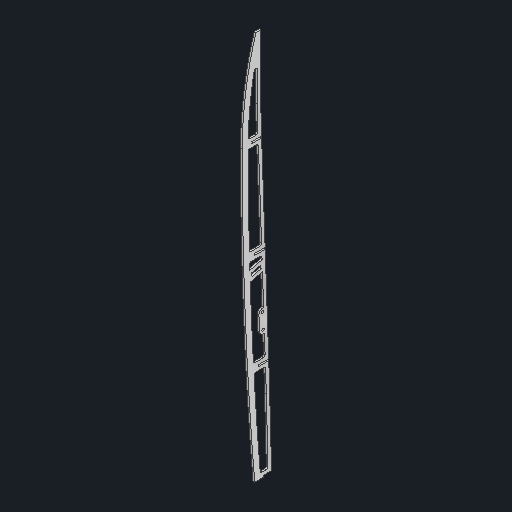
# Autodesk Inventor part: stringer_cowl
Saved by Autodesk Inventor 2023 (Build 270158030, 158C)
## iProperties
Created: 2022-03-23
Part Number: stringer_cowl
Material: Generic
Document SubType Name: Modeling
Designer: kardo
Density: 1 g/cm^3
Appearance: Default
Author: kardo
Autodesk Inventor part; units mm, degrees
ref_plane "YZ Plane" through (0, 0, 0) normal (1, 0, 0) x (0, 1, 0)
ref_plane "XZ Plane" through (0, 0, 0) normal (0, 1, 0) x (-1, 0, 0)
ref_plane "XY Plane" through (0, 0, 0) normal (0, 0, 1) x (1, 0, 0)
derived "parameters_frame.ipt"
derived "surface_body.ipt"
sketch "sk_rail_top_cowl" plane through (54.6, 0, 0) normal (1, 0, 0) x (0, 1, 0)
  spline S0 degree 2 poles (-345, 39.712) (-172.656, 54.3934) (0, 54.4) knots 0 0 0 1 1 1
  spline S1 degree 3 poles (0, 54.4) (37.026, 54.4) (80.784, 47.9917) (112.2, 37.536) knots 1 1 1 1 2 2 2 2
  point P0 (0, 0)
sketch "sk_rail_bottom_standoff" plane through (34.32, 0, 0) normal (1, 0, 0) x (0, 1, 0)
  line L0 (-345, 16.32) -> (-262.2001, 18.586)
  arc A0 (-262.2001, 18.586) -> (-241.5001, 19.2432) centre (-326.8578, 2381.2399) ccw
  line L1 (36.465, 28.832) -> (112.2, 28.832)
  arc A1 (36.465, 28.832) -> (11.22, 28.376) centre (36.465, -670.197) ccw
  line L2 (-241.5001, 19.2432) -> (11.22, 28.376)
  line L3 (-465, 0) -> (375, 0) construction
  line L4 (11.22, 28.376) -> (11.22, 0) construction
  line L5 (-241.5001, 19.2432) -> (-241.5001, 0) construction
  point P0 (0, 0)
  point P1 (-241.5001, 19.1524)
  point P2 (11.22, 28.832)
ref_plane "plane_middle" through (0, 0, 0) normal (0, 1, 0) x (-1, 0, 0)
ref_plane "plane_rear" through (0, -345, 0) normal (0, 1, 0) x (-1, 0, 0)
ref_plane "plane_cowl_right" through (54.6, 0, 0) normal (1, 0, 0) x (0, 1, 0)
ref_plane "plane_nose" through (0, 112.2, 0) normal (0, 1, 0) x (-1, 0, 0)
ref_plane "plane_tail_1" through (0, -114.9999, 0) normal (0, 1, 0) x (-1, 0, 0)
ref_plane "plane_tail_2" through (0, -230.0001, 0) normal (0, 1, 0) x (-1, 0, 0)
derived "stencil_frame.ipt"
sketch "sk_cowl_joint_locations" plane through (54.6, 0, 0) normal (1, 0, 0) x (0, 1, 0)
  line L0 (-345, 16.32) -> (-262.2001, 18.586) construction
  arc A0 (-262.2001, 18.586) -> (-241.5001, 19.2432) centre (-326.8578, 2381.2399) ccw construction
  line L1 (-241.5001, 19.2432) -> (11.22, 28.376) construction
  arc A1 (36.465, 28.832) -> (11.22, 28.376) centre (36.465, -670.197) ccw construction
  line L2 (36.465, 28.832) -> (112.2, 28.832) construction
  line L3 (94.8, 30.032) -> (36.465, 30.032) construction
  arc A2 (36.465, 30.032) -> (11.1767, 29.5752) centre (36.465, -670.197) ccw construction
  line L4 (11.1767, 29.5752) -> (-241.5434, 20.4424) construction
  arc A3 (-262.2329, 19.7855) -> (-241.5434, 20.4424) centre (-326.8578, 2381.2399) ccw construction
  line L5 (-262.2329, 19.7855) -> (-345, 17.5204) construction
  line L6 (-230.0001, 3089.1136) -> (-230.0001, -1866.0023) construction
  line L7 (-114.9999, 3089.1136) -> (-114.9999, -1866.0023) construction
  line L8 (-345, 3089.1136) -> (-345, -1866.0023) construction
  line L9 (0, 3089.1136) -> (0, -1866.0023) construction
  line L10 (-230.0001, 45.0685) -> (-230.0001, 20.8596) construction
  line L11 (-114.9999, 49.9659) -> (-114.9999, 25.0155) construction
  line L12 (-345, 17.5204) -> (-345, 17.5204)
  line L13 (-345, 17.5204) -> (-345, 36.9221) construction
  line L14 (-869.78, 3004.1953) -> (348.339, -1881.413) construction
  line L15 (-344.7623, 36.9221) -> (-345, 39.712) construction
  spline S0 degree 2 poles (-345, 39.712) (-172.656, 54.3934) (0, 54.4) knots 0 0 0 1 1 1
  spline S1 degree 3 poles (0, 54.4) (37.026, 54.4) (80.784, 47.9917) (112.2, 37.536) knots 1 1 1 1 2 2 2 2
  line L16 (0, 51.6) -> (0, 29.1713) construction
  spline S2 degree 3 poles (111.3158, 34.8793) (106.1488, 36.5989) (96.4909, 39.4217) (84.5445, 42.2265) (75.2974, 44.1359) (69.0059, 45.3094) (61.0256, 46.6466) (54.5653, 47.6105) (46.4371, 48.6777) (39.9092, 49.4192) (31.7597, 50.2005) (25.2653, 50.7072) (17.2211, 51.1873) (9.2717, 51.5118) (3.0586, 51.6) (0, 51.6) knots 1 1 1 1 1.166667 1.291667 1.333333 1.416667 1.458333 1.541667 1.583333 1.666667 1.708333 1.791667 1.833333 1.916667 2 2 2 2
  spline S3 degree 3 poles (0, 51.6) (-19.1708, 51.5993) (-52.7146, 51.3604) (-91.0402, 50.6121) (-119.7801, 49.8472) (-138.9379, 49.2354) (-162.8824, 48.3434) (-182.0358, 47.528) (-205.975, 46.3814) (-225.1241, 45.3623) (-249.0578, 43.9611) (-268.2026, 42.7383) (-292.131, 41.0825) (-316.0566, 39.2994) (-335.1942, 37.7372) (-344.7623, 36.9221) knots 0 0 0 0 0.166667 0.291667 0.333333 0.416667 0.458333 0.541666 0.583333 0.666666 0.708333 0.791666 0.833333 0.916666 1 1 1 1
  line L17 (-136.2088, 45.4676) -> (-130.9657, 24.4385) construction
  line L18 (-128.3953, 30.6635) -> (-132.2764, 29.6958) construction
  line L19 (-131.0168, 41.178) -> (-134.898, 40.2103) construction
  line L20 (-136.2088, 45.4676) -> (-132.3276, 46.4353) construction
  line L21 (-130.9657, 24.4385) -> (-127.0845, 25.4062) construction
  line L22 (-132.3276, 46.4353) -> (-132.5171, 52.2322) construction
  point P0 (0, 0)
  point P1 (-345, 27.2213)
  point P2 (-230.0001, 32.964)
  point P3 (-114.9999, 37.4907)
  point P4 (0, 40.3857)
  point P5 (-869.78, 3004.1953)
  point P6 (348.339, -1881.413)
  point P7 (-85.2629, 50.788)
  point P8 (0, 40.3857)
sketch "sk_servo_mount" plane through (-54.6, 0, 0) normal (1, 0, 0) x (0, 1, 0)
  line L0 (-241.5001, 19.2432) -> (11.22, 28.376) construction
  line L1 (-345, 3089.1136) -> (-345, -1866.0023) construction
  line L2 (0, 3089.1136) -> (0, -1866.0023) construction
  line L3 (-195.0558, 20.9216) -> (-195.2941, 27.5173) construction
  line L4 (-195.2941, 27.5173) -> (-177.3059, 28.1674) construction
  line L5 (-177.3059, 28.1674) -> (-177.0675, 21.5717) construction
  point P0 (0, 0)
  point P1 (-186.3, 27.8423)
sketch "sk_base" plane through (54.6, 0, 0) normal (1, 0, 0) x (0, 1, 0)
  line L0 (-345, 16.32) -> (-262.2001, 18.586) construction
  arc A0 (-262.2001, 18.586) -> (-241.5001, 19.2432) centre (-326.8578, 2381.2399) ccw construction
  line L1 (-241.5001, 19.2432) -> (11.22, 28.376) construction
  arc A1 (36.465, 28.832) -> (11.22, 28.376) centre (36.465, -670.197) ccw construction
  line L2 (36.465, 28.832) -> (112.2, 28.832) construction
  spline S0 degree 3 poles (0, 54.4) (37.026, 54.4) (80.784, 47.9917) (112.2, 37.536) knots 1 1 1 1 2 2 2 2 construction
  spline S1 degree 2 poles (-345, 39.712) (-172.656, 54.3934) (0, 54.4) knots 0 0 0 1 1 1 construction
  line L3 (-345, 4592.9714) -> (-345, -1605.7041) projected
  line L4 (112.2, 4592.9714) -> (112.2, -1605.7041) construction
  line L5 (110.2, 30.032) -> (36.465, 30.032)
  arc A2 (36.465, 30.032) -> (11.1767, 29.5752) centre (36.465, -670.197) ccw
  line L6 (11.1767, 29.5752) -> (-241.5434, 20.4424)
  arc A3 (-262.2329, 19.7855) -> (-241.5434, 20.4424) centre (-326.8578, 2381.2399) ccw
  line L7 (-262.2329, 19.7855) -> (-345.0328, 17.5196)
  line L8 (110.2, 35.668) -> (110.2, 30.032)
  line L9 (-345, 39.712) -> (-344.7963, 37.3207) construction
  line L10 (-344.7963, 37.3207) -> (-345, 37.3033)
  spline S2 degree 4 poles (-344.7963, 37.3207) (-258.8046, 44.646) (-172.6063, 49.5475) (-86.303, 51.9967) (0.0001, 52) knots 0 0 0 0 0 1 1 1 1 1
  spline S3 degree 5 poles (0, 52) (11.6151, 51.9997) (23.2289, 51.4722) (34.8145, 50.543) (57.0458, 48.0136) (79.0573, 44.0004) (89.562, 41.7015) (99.982, 38.9984) (110.2, 35.6678) knots 0 0 0 0 0 0 0.519409 0.519409 0.519409 1 1 1 1 1 1
  point P0 (0, 0)
  point P1 (-345, 17.5204)
  dimension "d3" = 2.4
  dimension "d2" = 1.2
  dimension "d4" = 2
  constraints: 12 end point, 4 point on circle, 2 centre point, 1 parallel, 1 perpendicular, 1 point on line, 12 other
  measures "d2" distance between parallel lines of L1 L6
  measures "d4" distance between parallel lines of L4 L8
extrude "thicken" add sketch "sk_base" along normal blind 2
sketch "sk_cut_weight" plane through (54.6, 0, 0) normal (1, 0, 0) x (0, 1, 0)
  spline S0 degree 3 poles (-344.7963, 37.3207) (-335.2272, 38.1358) (-316.0877, 39.6982) (-292.1597, 41.4815) (-268.2291, 43.1374) (-249.0824, 44.3603) (-225.1463, 45.7617) (-205.9953, 46.7809) (-182.0538, 47.9276) (-162.8984, 48.7431) (-138.9516, 49.6352) (-119.7919, 50.247) (-95.8396, 50.8845) (-76.6756, 51.2926) (-52.7179, 51.6755) (-28.7575, 51.931) (-9.5863, 51.9996) (0, 52) knots 0 0 0 0 0.083333 0.166667 0.208333 0.291667 0.333333 0.416667 0.458333 0.541667 0.583333 0.666667 0.708333 0.791667 0.833333 0.916667 1 1 1 1 construction
  line L0 (-262.2329, 19.7855) -> (-345.0328, 17.5196) construction
  line L1 (110.2, 35.668) -> (110.2, 30.032) construction
  line L2 (-114.9999, 4592.9714) -> (-114.9999, -1605.7041) construction
  line L3 (-230.0001, 4592.9714) -> (-230.0001, -1605.7041) construction
  line L4 (-345, 4592.9714) -> (-345, -1605.7041) construction
  line L5 (0, 4592.9714) -> (0, -1605.7041) construction
  line L6 (11.1767, 29.5752) -> (-241.5434, 20.4424) construction
  arc A0 (-262.2329, 19.7855) -> (-241.5434, 20.4424) centre (-326.8578, 2381.2399) ccw construction
  line L7 (110.2, 30.032) -> (36.465, 30.032) construction
  arc A1 (36.465, 30.032) -> (11.1767, 29.5752) centre (36.465, -670.197) ccw construction
  spline S1 degree 3 poles (0, 52) (3.0219, 52) (9.1586, 51.914) (17.0078, 51.5976) (24.9501, 51.1295) (31.3623, 50.6354) (39.4099, 49.8733) (45.8578, 49.1499) (53.8895, 48.1087) (60.2761, 47.168) (68.1706, 45.8627) (74.3991, 44.7169) (82.0351, 43.1629) (88.0081, 41.8244) (95.2639, 40.0376) (102.2888, 38.1399) (107.6186, 36.5095) (110.2, 35.668) knots 1 1 1 1 1.082229 1.164457 1.205571 1.2878 1.328914 1.411142 1.452257 1.534485 1.575599 1.657828 1.698942 1.78117 1.822284 1.904513 1.986741 1.986741 1.986741 1.986741 construction
  line L8 (-343, 17.5196) -> (-343, 52) construction
  line L9 (-228.0001, 52) -> (-228.0001, 17.5196) construction
  line L10 (-112.9999, 52) -> (-112.9999, 17.5196) construction
  line L11 (2, 52) -> (2, 17.5196) construction
  line L12 (-339, 30.7857) -> (-339, 21.6861)
  line L13 (-234.0001, 24.7176) -> (-234.0001, 38.2283)
  line L14 (-224.0001, 38.7947) -> (-224.0001, 25.079)
  line L15 (-108.9999, 43.5294) -> (-108.9999, 29.2349)
  line L16 (-4, 33.0294) -> (-4, 44.9979)
  line L17 (6, 44.9437) -> (6, 33.3908)
  line L18 (90.3642, 34.032) -> (36.465, 34.032)
  arc A2 (36.465, 34.032) -> (11.0322, 33.5726) centre (36.465, -670.197) ccw
  line L19 (11.0322, 33.5726) -> (-241.6879, 24.4398)
  arc A3 (-262.3423, 23.784) -> (-241.6879, 24.4398) centre (-326.8578, 2381.2399) ccw
  line L20 (-262.3423, 23.784) -> (-343, 21.5767)
  line L21 (-118.9999, 43.2475) -> (-118.9999, 28.8735)
  spline S2 degree 5 poles (90.3642, 34.0321) (83.5768, 35.7135) (76.7406, 37.198) (69.8723, 38.519) (51.8764, 41.5622) (33.7339, 43.6027) (22.5075, 44.4934) (11.2545, 44.9997) (0, 45) knots 0 0 0 0 0 0 0.383219 0.383219 0.383219 1 1 1 1 1 1
  spline S3 degree 4 poles (0.0003, 45) (-85.8525, 44.9967) (-171.7055, 42.5688) (-257.4548, 37.7099) (-343, 30.4481) knots 0 0 0 0 0 1 1 1 1 1
  point P0 (0, 0)
  dimension "d51" = 7
  dimension "d18" = 2
  dimension "d19" = 2
  dimension "d20" = 2
  dimension "d21" = 2
  dimension "d22" = 4
  dimension "d23" = 4
  dimension "d26" = 4
  dimension "d27" = 4
  dimension "d28" = 4
  dimension "d29" = 4
  dimension "d30" = 4
  dimension "d52" = 4
  constraints: 28 end point, 11 parallel, 9 point on line, 8 horizontal alignment, 4 point on circle, 2 centre point, 17 other
  measures "d18" distance between parallel lines of L3 L9
  measures "d19" distance between parallel lines of L10 L2
  measures "d20" distance between parallel lines of L11 L5
  measures "d21" distance between parallel lines of L8 L4
  measures "d22" distance between parallel lines of L8 L12
  measures "d23" distance between parallel lines of L13 L3
  measures "d26" distance between parallel lines of L9 L14
  measures "d27" distance between parallel lines of L10 L15
  measures "d28" distance between parallel lines of L16 L5
  measures "d29" distance between parallel lines of L11 L17
  measures "d30" distance between parallel lines of L21 L2
  measures "d52" distance between parallel lines of L7 L18
extrude "cut_weight" cut sketch "sk_cut_weight" along normal through all both and the other way through all contours S3 L13 L19 A3 L20 L12 | S3 L21 L19 L14 | S3 L16 L19 L15 | L17 S2 L18 A2 L19
fillet "rounding" radius 2 15 edges at (55.6, -234.0001, 24.7176) (55.6, -118.9999, 28.8735) (55.6, -4, 33.0294) (55.6, 6, 33.3908) (55.6, -108.9999, 29.2349) (55.6, -224.0001, 25.079) (55.6, -339, 21.6861) (55.6, -339, 30.7857) (55.6, -224.0001, 38.7947) (55.6, -108.9999, 43.5294) (55.6, 6, 44.9437) (55.6, -4, 44.9979) (55.6, -118.9999, 43.2475) (55.6, -234.0001, 38.2283) (55.6, 90.3642, 34.032)
sketch "sk_joint_motor_mount" plane through (54.6, 0, 0) normal (1, 0, 0) x (0, 1, 0)
  spline S0 degree 3 poles (-344.7963, 37.3207) (-335.2272, 38.1358) (-316.0877, 39.6982) (-292.1597, 41.4815) (-268.2291, 43.1374) (-249.0824, 44.3603) (-225.1463, 45.7617) (-205.9953, 46.7809) (-182.0538, 47.9276) (-162.8984, 48.7431) (-138.9516, 49.6352) (-119.7919, 50.247) (-95.8396, 50.8845) (-76.6756, 51.2926) (-52.7179, 51.6755) (-28.7575, 51.931) (-9.5863, 51.9996) (0, 52) knots 0 0 0 0 0.083333 0.166667 0.208333 0.291667 0.333333 0.416667 0.458333 0.541667 0.583333 0.666667 0.708333 0.791667 0.833333 0.916667 1 1 1 1 projected
  line L0 (11.1767, 29.5752) -> (-241.5434, 20.4424) projected
  line L1 (-131.0168, 41.178) -> (-128.3953, 30.6635) construction
  line L2 (-131.0168, 41.178) -> (-134.898, 40.2103) construction
  line L3 (-134.898, 40.2103) -> (-132.2764, 29.6958) construction
  line L4 (-132.2764, 29.6958) -> (-128.3953, 30.6635) construction
  line L5 (-141.3448, 49.5326) -> (-135.0513, 24.2908)
  line L6 (-129.0795, 49.9419) -> (-122.7944, 24.7338)
  point P0 (0, 0)
  dimension "d33" = 4
  dimension "d34" = 4
  dimension "d35" = 4
  constraints: 12 end point, 3 parallel, 2 coincident, 2 perpendicular, 2 point on line, 2 other
  measures "d33" distance between parallel lines of L1 L3
  measures "d34" distance between parallel lines of L3 L5
  measures "d35" distance between parallel lines of L1 L6
extrude "joint_motor_mount" add sketch "sk_joint_motor_mount" along normal blind 2
sketch "sk_joint_servo" plane through (54.6, 0, 0) normal (1, 0, 0) x (0, 1, 0)
  line L0 (11.1767, 29.5752) -> (-241.5434, 20.4424) projected
  line L1 (-171.8973, 22.9593) -> (-173.1987, 29.0456)
  arc A0 (-173.1987, 29.0456) -> (-177.4576, 32.3646) centre (-177.3059, 28.1674) ccw
  line L2 (-177.4576, 32.3646) -> (-195.4458, 31.7146)
  arc A1 (-195.4458, 31.7146) -> (-199.454, 28.0968) centre (-195.2941, 27.5173) ccw
  line L3 (-199.454, 28.0968) -> (-200.3127, 21.9324)
  point P0 (0, 0)
  dimension "d39" = 80
  dimension "d40" = 80
  dimension "d41" = 4.2
  constraints: 6 end point, 4 point on circle, 4 tangent, 2 centre point, 2 coincident, 2 point on line, 1 equal radius
  measures "d39" angle of L1 L0
  measures "d40" angle of L0 L3
  measures "d41" radius of A0
extrude "joint_servo" add sketch "sk_joint_servo" along normal blind 2
hole "drill_joint_servo" at (54.6, -195.2941, 27.5173) at (54.6, -177.3059, 28.1674) direction (1, 0, 0) diameter 3 end through all
sketch "sk_cowl_joint_cuts" plane through (54.6, 0, 0) normal (1, 0, 0) x (0, 1, 0)
  line L0 (-230.0001, 2991.5273) -> (-230.0001, -1280.4843) projected
  line L1 (-114.9999, 2991.5273) -> (-114.9999, -1280.4843) projected
  line L2 (0, 2991.5273) -> (0, -1280.4843) projected
  line L3 (-345, 2991.5273) -> (-345, -1280.4843) projected
  line L4 (-114.9999, -12.5093) -> (-112.9999, -12.5093)
  line L5 (-112.9999, -12.5093) -> (-112.9999, 37.4907)
  line L6 (-112.9999, 37.4907) -> (-114.9999, 37.4907)
  line L7 (0, -9.6143) -> (2, -9.6143)
  line L8 (2, -9.6143) -> (2, 40.3857)
  line L9 (2, 40.3857) -> (0, 40.3857)
  line L10 (-230.0001, 32.964) -> (-228.0001, 32.964)
  line L11 (-228.0001, 32.964) -> (-228.0001, -17.036)
  line L12 (-228.0001, -17.036) -> (-230.0001, -17.036)
  line L13 (-345, 27.2213) -> (-343, 27.2213)
  line L14 (-343, 27.2213) -> (-343, -22.7787)
  line L15 (-343, -22.7787) -> (-345, -22.7787)
  line L16 (-128.3953, 30.6635) -> (-131.0168, 41.178)
  line L17 (-131.0168, 41.178) -> (-134.898, 40.2103)
  line L18 (-134.898, 40.2103) -> (-132.2764, 29.6958)
  line L19 (-132.2764, 29.6958) -> (-128.3953, 30.6635)
  point P0 (0, 0)
  dimension "d8" = 2
  dimension "d15" = 50
  dimension "d16" = 4
  constraints: 33 end point, 11 parallel, 10 perpendicular, 4 point on line
  measures "d8" distance of L8.end L9.end
  measures "d15" distance of L7.end L8.end
  measures "d16" distance of L16.end L17.end
extrude "cut_joints" cut sketch "sk_cowl_joint_cuts" along normal through all
equation "\"d2\" = shell_thickness"
equation "\"d5\" = bulkhead_thickness"
equation "\"d51\" = bulkhead_inset + cowl_sealing_thickness"
equation "\"d18\" = bulkhead_thickness"
equation "\"d19\" = bulkhead_thickness"
equation "\"d20\" = bulkhead_thickness"
equation "\"d21\" = bulkhead_thickness"
equation "\"d22\" = bulkhead_inset"
equation "\"d23\" = bulkhead_inset"
equation "\"d26\" = bulkhead_inset"
equation "\"d27\" = bulkhead_inset"
equation "\"d28\" = bulkhead_inset"
equation "\"d29\" = bulkhead_inset"
equation "\"d30\" = bulkhead_inset"
equation "\"d38\" = 0.5 * bulkhead_inset"
equation "\"d33\" = 2 * bulkhead_thickness"
equation "\"d34\" = bulkhead_inset"
equation "\"d35\" = bulkhead_inset"
equation "\"d36\" = bulkhead_thickness"
equation "\"d41\" = 1.4 * drill_servo_mount_diam"
equation "\"d42\" = bulkhead_thickness"
equation "\"d44\" = drill_servo_mount_diam"
equation "\"d8\" = bulkhead_thickness"
equation "\"d16\" = 2 * bulkhead_thickness"
equation "\"shell_thickness\" = 1.2"
equation "\"bulkhead_thickness\" = 2"
equation "\"bulkhead_inset\" = 4"
equation "\"cowl_sealing_thickness\" = 3"
equation "\"drill_servo_mount_diam\" = 3"
body "Solid1"
